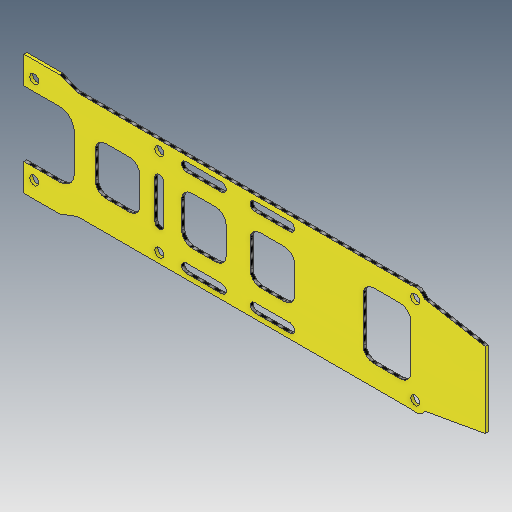
# Autodesk Inventor part: Top Plate
Saved by Autodesk Inventor 2018 (Build 220112000, 112)
## iProperties
Created: 2018-01-03
Part Number: Top Plate
Material: CFRP
Document SubType Name: Modeling
Designer: fbl92568
Mass: 5.50135 g
Surface Area: 85.6738 cm^2
Volume: 3.8471 cm^3
Density: 1.43 g/cm^3
Appearance: Carbon Fiber
Author: fbl92568
Autodesk Inventor part; units mm, degrees
ref_plane "YZ Plane" through (0, 0, 0) normal (1, 0, 0) x (0, 1, 0)
ref_plane "XZ Plane" through (0, 0, 0) normal (0, 1, 0) x (-1, 0, 0)
ref_plane "XY Plane" through (0, 0, 0) normal (0, 0, 1) x (1, 0, 0)
sketch "Sketch1" plane through (0, 0, 0) normal (0, 0, 1) x (1, 0, 0)
  line L0 (-74, 14.75) -> (54, 14.75) construction
  line L1 (-89.2201, 0) -> (135.4294, 0) construction
  circle A0 centre (-74, 14.75) radius 1.525
  circle A1 centre (-32, 14.75) radius 1.525
  circle A2 centre (54, 14.75) radius 1.525
  line L2 (-77.5, 0.7411) -> (-77.5, 20.25)
  line L3 (-77.5, 20.25) -> (77.5, 20.25)
  line L4 (77.5, 20.25) -> (77.5, 0)
  line L5 (-74, -14.75) -> (54, -14.75) construction
  circle A3 centre (-74, -14.75) radius 1.525
  circle A4 centre (-32, -14.75) radius 1.525
  circle A5 centre (54, -14.75) radius 1.525
  line L6 (-77.5, -0.7411) -> (-77.5, -20.25)
  line L7 (-77.5, -20.25) -> (77.5, -20.25)
  line L8 (77.5, -20.25) -> (77.5, 0)
  line L9 (-77.5, 0.7411) -> (-77.5, -0.7411)
  point P0 (0, 0)
  point P1 (0, 0)
  dimension "d2" = 3.05
  dimension "d3" = 3.05
  dimension "d4" = 3.05
  dimension "d6" = 42
  dimension "d7" = 86
  dimension "d127" = 20.25
  dimension "d129" = 155
  dimension "d130" = 77.5
  dimension "d131" = 3.5
  constraints: 20 end point, 8 symmetric about line, 6 centre point, 6 coincident, 4 point on line, 1 horizontal, 1 parallel, 1 vertical, 3 other
  measures "d2" diameter of A0
  measures "d3" diameter of A1
  measures "d4" diameter of A2
  measures "d6" distance of A1.centre A0.centre
  measures "d7" distance of A2.centre A1.centre
  measures "d127" distance from line of point (0, 0) L3
  measures "d129" distance of L2.end L3.end
  measures "d130" distance from line of point (0, 0) L4
  measures "d131" distance from line of L2 A0.centre
extrude "Extrusion1" add sketch "Sketch1" along normal blind 1
sketch "Sketch5" plane through (0, 0, 1) normal (0, 0, 1) x (1, 0, 0)
  line L0 (-59.5, -18) -> (-65.5, -20.25)
  line L1 (-77.5, -11) -> (-65.5, -11)
  line L2 (0, 40.5196) -> (0, -40.5196) projected
  line L3 (-109.7892, 0) -> (116.2355, 0) projected
  line L4 (-60.5, -6) -> (-60.5, 0)
  arc A0 (-65.5, -11) -> (-60.5, -6) centre (-65.5, -6) ccw
  circle A1 centre (54, -14.75) radius 1.525 projected
  arc A2 (52.701, -18) -> (57.1503, -16.275) centre (54, -14.75) ccw
  line L5 (52.701, -18) -> (-59.5, -18)
  line L6 (57.1503, -16.275) -> (77.5, -12.6734)
  arc A3 (57.1503, -16.275) -> (52.701, -18) centre (54, -14.75) ccw construction
  line L7 (49, -11) -> (40, -11)
  line L8 (36.5, -7.5) -> (36.5, 0)
  line L9 (52.5, 0) -> (52.5, -7.5)
  line L10 (-42, -8) -> (-50, -8)
  line L11 (-53.5, -4.5) -> (-53.5, 0)
  line L12 (-38.5, 0) -> (-38.5, -4.5)
  line L13 (-30.5, 0) -> (-30.5, -6.5)
  line L14 (-33.5, -6.5) -> (-33.5, 0)
  arc A4 (-33.5, -6.5) -> (-30.5, -6.5) centre (-32, -6.5) ccw
  line L15 (-9.5, 0) -> (-9.5, -4.5)
  line L16 (-13, -8) -> (-21, -8)
  line L17 (-24.5, -4.5) -> (-24.5, 0)
  line L18 (10, -8) -> (2, -8)
  line L19 (-1.5, -4.5) -> (-1.5, 0)
  line L20 (13.5, 0) -> (13.5, -4.5)
  circle A5 centre (-32, -14.75) radius 1.525 construction
  line L21 (-32, -14.75) -> (15.7139, -14.75) construction
  circle A6 centre (-32, 14.75) radius 1.525 construction
  line L22 (-32, 14.75) -> (13.5, 14.75) construction
  line L23 (12, -28.9426) -> (12, 23.2337) construction
  line L24 (0, -27.2548) -> (0, 23.7474) construction
  line L25 (-11, -24.7597) -> (-11, 23.7474) construction
  line L26 (-23, -24.7597) -> (-23, 23.7474) construction
  line L27 (12, -14.75) -> (0, -14.75) construction
  line L28 (12, -13.25) -> (0, -13.25)
  line L29 (0, -16.25) -> (12, -16.25)
  arc A7 (12, -16.25) -> (12, -13.25) centre (12, -14.75) ccw
  arc A8 (0, -13.25) -> (0, -16.25) centre (0, -14.75) ccw
  line L30 (-11, -14.75) -> (-23, -14.75) construction
  line L31 (-11, -13.25) -> (-23, -13.25)
  line L32 (-23, -16.25) -> (-11, -16.25)
  arc A9 (-11, -16.25) -> (-11, -13.25) centre (-11, -14.75) ccw
  arc A10 (-23, -13.25) -> (-23, -16.25) centre (-23, -14.75) ccw
  arc A11 (49, -11) -> (52.5, -7.5) centre (49, -7.5) ccw
  arc A12 (36.5, -7.5) -> (40, -11) centre (40, -7.5) ccw
  arc A13 (10, -8) -> (13.5, -4.5) centre (10, -4.5) ccw
  arc A14 (-1.5, -4.5) -> (2, -8) centre (2, -4.5) ccw
  arc A15 (-13, -8) -> (-9.5, -4.5) centre (-13, -4.5) ccw
  arc A16 (-24.5, -4.5) -> (-21, -8) centre (-21, -4.5) ccw
  arc A17 (-42, -8) -> (-38.5, -4.5) centre (-42, -4.5) ccw
  arc A18 (-53.5, -4.5) -> (-50, -8) centre (-50, -4.5) ccw
  line L33 (-59.5, 18) -> (-65.5, 20.25)
  line L34 (-77.5, 11) -> (-65.5, 11)
  line L35 (-60.5, 6) -> (-60.5, 0)
  arc A19 (-60.5, 6) -> (-65.5, 11) centre (-65.5, 6) ccw
  circle A20 centre (54, 14.75) radius 1.525
  arc A21 (57.1503, 16.275) -> (52.701, 18) centre (54, 14.75) ccw
  line L36 (52.701, 18) -> (-59.5, 18)
  line L37 (57.1503, 16.275) -> (77.5, 12.6734)
  arc A22 (52.701, 18) -> (57.1503, 16.275) centre (54, 14.75) ccw construction
  line L38 (49, 11) -> (40, 11)
  line L39 (36.5, 7.5) -> (36.5, 0)
  line L40 (52.5, 0) -> (52.5, 7.5)
  line L41 (-42, 8) -> (-50, 8)
  line L42 (-53.5, 4.5) -> (-53.5, 0)
  line L43 (-38.5, 0) -> (-38.5, 4.5)
  line L44 (-30.5, 0) -> (-30.5, 6.5)
  line L45 (-33.5, 6.5) -> (-33.5, 0)
  arc A23 (-30.5, 6.5) -> (-33.5, 6.5) centre (-32, 6.5) ccw
  line L46 (-9.5, 0) -> (-9.5, 4.5)
  line L47 (-13, 8) -> (-21, 8)
  line L48 (-24.5, 4.5) -> (-24.5, 0)
  line L49 (10, 8) -> (2, 8)
  line L50 (-1.5, 4.5) -> (-1.5, 0)
  line L51 (13.5, 0) -> (13.5, 4.5)
  circle A24 centre (-32, 14.75) radius 1.525 construction
  line L52 (-32, 14.75) -> (15.7139, 14.75) construction
  line L53 (12, 14.75) -> (0, 14.75) construction
  line L54 (12, 13.25) -> (0, 13.25)
  line L55 (0, 16.25) -> (12, 16.25)
  arc A25 (12, 13.25) -> (12, 16.25) centre (12, 14.75) ccw
  arc A26 (0, 16.25) -> (0, 13.25) centre (0, 14.75) ccw
  line L56 (-11, 14.75) -> (-23, 14.75) construction
  line L57 (-11, 13.25) -> (-23, 13.25)
  line L58 (-23, 16.25) -> (-11, 16.25)
  arc A27 (-11, 13.25) -> (-11, 16.25) centre (-11, 14.75) ccw
  arc A28 (-23, 16.25) -> (-23, 13.25) centre (-23, 14.75) ccw
  arc A29 (52.5, 7.5) -> (49, 11) centre (49, 7.5) ccw
  arc A30 (40, 11) -> (36.5, 7.5) centre (40, 7.5) ccw
  arc A31 (13.5, 4.5) -> (10, 8) centre (10, 4.5) ccw
  arc A32 (2, 8) -> (-1.5, 4.5) centre (2, 4.5) ccw
  arc A33 (-9.5, 4.5) -> (-13, 8) centre (-13, 4.5) ccw
  arc A34 (-21, 8) -> (-24.5, 4.5) centre (-21, 4.5) ccw
  arc A35 (-38.5, 4.5) -> (-42, 8) centre (-42, 4.5) ccw
  arc A36 (-50, 8) -> (-53.5, 4.5) centre (-50, 4.5) ccw
  line L59 (77.5, -12.6734) -> (82.2803, -14.75)
  line L60 (82.2803, -14.75) -> (77.5, -28.9426)
  line L61 (77.5, -28.9426) -> (-65.5, -24.3901)
  line L62 (-65.5, -24.3901) -> (-65.5, -20.25)
  line L63 (77.5, 12.6734) -> (83.9462, 22.4701)
  line L64 (83.9462, 22.4701) -> (-65.5, 21.6624)
  line L65 (-65.5, 21.6624) -> (-65.5, 20.25)
  line L66 (-77.5, -11) -> (-77.5, 11)
  point P0 (0, 0)
  point P1 (-77.5, -20.25)
  point P2 (-77.5, 20.25)
  point P3 (52.5, -11)
  point P4 (36.5, -11)
  point P5 (-38.5, -8)
  point P6 (-53.5, -8)
  point P7 (-9.5, -8)
  point P8 (-24.5, -8)
  point P9 (-1.5, -8)
  point P10 (6, -14.75)
  point P11 (-17, -14.75)
  point P12 (52.5, 11)
  point P13 (36.5, 11)
  point P14 (-38.5, 8)
  point P15 (-53.5, 8)
  point P16 (-9.5, 8)
  point P17 (-24.5, 8)
  point P18 (-1.5, 8)
  point P19 (12, 28.9426)
  point P20 (0, 27.2548)
  point P21 (-11, 24.7597)
  point P22 (-23, 24.7597)
  point P23 (6, 14.75)
  point P24 (-17, 14.75)
  dimension "d133" = 12
  dimension "d135" = 11
  dimension "d137" = 5
  dimension "d138" = 7
  dimension "d139" = 97
  dimension "d140" = 16
  dimension "d141" = 8
  dimension "d142" = 7
  dimension "d143" = 15
  dimension "d144" = 3
  dimension "d147" = 6.5
  dimension "d148" = 15
  dimension "d149" = 8
  dimension "d150" = 36
  dimension "d151" = 15
  dimension "d152" = 8
  dimension "d153" = 59
  dimension "d154" = 27
  dimension "d155" = 6.5
  dimension "d156" = 1.5
  dimension "d157" = 1.5
  dimension "d158" = 1.5
  dimension "d159" = 1.5
  dimension "d161" = 3.5
  constraints: 138 end point, 64 point on circle, 64 symmetric about line, 46 point on line, 34 centre point, 26 tangent, 7 equal radius, 7 parallel, 6 horizontal, 5 perpendicular, 4 vertical, 2 coincident, 2 midpoint, 18 other
  measures "d133" distance of point (-77.5, -20.25) L0.end
  measures "d135" distance from line of point (0, 0) L1
  measures "d137" radius of A0
  measures "d138" diameter of A2
  measures "d139" distance between parallel lines of L8 L4
  measures "d140" distance of point (52.5, -11) point (36.5, -11)
  measures "d141" distance of point (-53.5, -8) L11.end
  measures "d142" distance between parallel lines of L11 L4
  measures "d143" distance of point (-38.5, -8) point (-53.5, -8)
  measures "d144" distance of L13.end L14.start
  measures "d147" distance of L13.start L13.end
  measures "d148" distance of point (-9.5, -8) point (-24.5, -8)
  measures "d149" distance of L15.start point (-9.5, -8)
  measures "d150" distance between parallel lines of L4 L17
  measures "d151" distance of L19.end L20.start
  measures "d152" distance of point (-1.5, -8) L19.end
  measures "d153" distance between parallel lines of L4 L19
  measures "d154" distance between parallel lines of L4 L14
  measures "d155" distance of L14.start L14.end
  measures "d156" distance between parallel lines of L17 L26
  measures "d157" distance between parallel lines of L15 L25
  measures "d158" distance between parallel lines of L19 L24
  measures "d159" distance between parallel lines of L20 L23
  measures "d161" radius of A11
extrude "Extrusion5" cut sketch "Sketch5" against normal through all contours L5 L2 L61 L62 L0 | L4 A0 L1 L66 L3 | L3 L66 L34 A19 L35 | L12 A17 L10 A18 L11 L3 | L3 L42 A36 L41 A35 L43 | L13 A4 L14 L3 | L3 L45 A23 L44 | L15 A15 L16 A16 L17 L3 | L3 L48 A34 L47 A33 L46 | L36 L33 L65 L64 L2 | L2 L64 L63 L37 A21 L36 | A26 L2 | L2 L55 A25 L54 | L39 A30 L38 A29 L40 L3 | L3 L9 A11 L7 A12 L8 | A14 L19 L3 L2 | L2 L3 L20 A13 L18 A14 | A8 L2 | L2 L28 A7 L29 | L5 A2 L6 L59 L60 L61 L2 | L3 L50 A32 L2 | L2 A32 L49 A31 L51 L3 | A9 L32 A10 L31 | L57 A28 L58 A27
equation "\"d3\" = d2"
equation "\"d4\" = d2"
body "Solid1"
